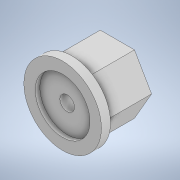
# Autodesk Inventor part: SpoolClutchFixedPlate
Saved by Autodesk Inventor 2020.2 (Build 242310000, 310)
## iProperties
Created: 2020-09-21
Part Number: SpoolClutchFixedPlate
Material: Generic
Document SubType Name: Modeling
Designer: elmar
Density: 1 g/cm^3
Appearance: Default
Author: elmar
Autodesk Inventor part; units mm, degrees
ref_plane "YZ Plane" through (0, 0, 0) normal (1, 0, 0) x (0, 1, 0)
ref_plane "XZ Plane" through (0, 0, 0) normal (0, 1, 0) x (-1, 0, 0)
ref_plane "XY Plane" through (0, 0, 0) normal (0, 0, 1) x (1, 0, 0)
sketch "Sketch1" plane through (0, 0, 0) normal (0, 0, 1) x (1, 0, 0)
  circle A0 centre (0, 0) radius 8.5
  dimension "d0" = 17
  constraints: 1 centre point, 1 coincident
  measures "d0" diameter of A0
extrude "Extrusion1" add sketch "Sketch1" along normal blind 10
sketch "Sketch4" plane through (0, 0, 10) normal (0, 0, 1) x (1, 0, 0)
  circle A0 centre (0, 0) radius 8.5 projected
extrude "Extrusion4" add sketch "Sketch4" along normal blind 2
sketch "Sketch5" plane through (0, 0, 12) normal (0, 0, 1) x (1, 0, 0)
  point P0 (0, 0)
hole "Hole1" at (0, 0, 12) direction (0, 0, -1) diameter 3.2 end through all counterbore diameter 12 counterbore depth 1 clearance for "Socket Head Cap Screw" size "M3" standard "Ansi Metric M Profile"
sketch "Sketch9" plane through (0, 0, 0) normal (0, 0, -1) x (-1, 0, 0)
  line L0 (-3.7528, 6.5) -> (3.7528, 6.5)
  line L1 (3.7528, 6.5) -> (7.5056, 0)
  line L2 (7.5056, 0) -> (3.7528, -6.5)
  line L3 (3.7528, -6.5) -> (-3.7528, -6.5)
  line L4 (-3.7528, -6.5) -> (-7.5056, 0)
  line L5 (-7.5056, 0) -> (-3.7528, 6.5)
  circle A0 centre (0, 0) radius 8.5 projected
  dimension "d27" = 13
  constraints: 12 end point, 1 coincident, 1 horizontal, 13 other
  measures "d27" distance between parallel lines of L3 L0
extrude "Extrusion8" cut sketch "Sketch9" against normal blind 10
sketch "Sketch3" plane through (0, 0, 0) normal (0, 0, 1) x (1, 0, 0)
  line L0 (-1.5588, 2.7) -> (1.5588, 2.7)
  line L1 (1.5588, 2.7) -> (3.1177, 0)
  line L2 (3.1177, 0) -> (1.5588, -2.7)
  line L3 (1.5588, -2.7) -> (-1.5588, -2.7)
  line L4 (-1.5588, -2.7) -> (-3.1177, 0)
  line L5 (-3.1177, 0) -> (-1.5588, 2.7)
  point P0 (0, 0)
  point P1 (0, 0)
  dimension "d6" = 5.4
  constraints: 12 end point, 1 coincident, 1 horizontal, 13 other
  measures "d6" distance between parallel lines of L3 L0
extrude "Extrusion3" cut sketch "Sketch3" along normal blind 8
body "Solid1"
